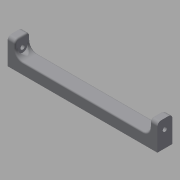
# Autodesk Inventor part: SwarmieLidSupport
Saved by Autodesk Inventor 2014 (Build 180170000, 170)
## iProperties
Created: 2015-05-25
Part Number: SwarmieLidSupport
Material: Generic
Document SubType Name: Modeling
Designer: Karl
Density: 1 g/cm^3
Appearance: Default
Author: Karl
Autodesk Inventor part; units mm, degrees
ref_plane "YZ Plane" through (0, 0, 0) normal (1, 0, 0) x (0, 1, 0)
ref_plane "XZ Plane" through (0, 0, 0) normal (0, 1, 0) x (-1, 0, 0)
ref_plane "XY Plane" through (0, 0, 0) normal (0, 0, 1) x (1, 0, 0)
sketch "Sketch1" plane through (0, 0, 0) normal (0, 1, 0) x (-1, 0, 0)
  line L0 (63.5, -6.35) -> (-63.5, -6.35)
  line L1 (-63.5, -6.35) -> (-63.5, 6.35)
  line L2 (-63.5, 6.35) -> (63.5, 6.35)
  line L3 (63.5, 6.35) -> (63.5, -6.35)
  line L4 (63.5, -6.35) -> (-63.5, 6.35) construction
  line L5 (-63.5, -6.35) -> (63.5, 6.35) construction
  point P0 (0, 0)
  dimension "d0" = 12.7
  dimension "d1" = 127
  constraints: 12 end point, 2 midpoint, 2 parallel, 1 horizontal, 1 perpendicular
  measures "d0" distance of L0.end L1.end
  measures "d1" distance of L1.end L2.end
extrude "Extrusion1" add sketch "Sketch1" along normal blind 22.225
sketch "Sketch2" plane through (-63.5, 0, 6.35) normal (0, 0, 1) x (1, 0, 0)
  line L0 (127, 0) -> (0, 0) projected
  line L1 (127, 0) -> (127, 22.225) projected
  line L2 (0, 22.225) -> (127, 22.225) projected
  line L3 (0, 0) -> (0, 22.225) projected
  line L4 (6.35, 22.225) -> (120.65, 22.225)
  line L5 (120.65, 22.225) -> (120.65, 9.525)
  line L6 (120.65, 9.525) -> (6.35, 9.525)
  line L7 (6.35, 9.525) -> (6.35, 22.225)
  point P0 (63.5, 0)
  dimension "d4" = 6.35
  dimension "d5" = 6.35
  dimension "d6" = 9.525
  constraints: 8 end point, 2 parallel, 1 horizontal, 1 perpendicular, 1 point on line
  measures "d4" distance between parallel lines of L3 L7
  measures "d5" distance between parallel lines of L1 L5
  measures "d6" distance between parallel lines of L0 L6
extrude "Extrusion2" cut sketch "Sketch2" against normal blind 22.225 contours L5 L6 L7 L2
fillet "Fillet1" radius 6.35 2 edges at (57.15, 9.525, 0) (-57.15, 9.525, 0)
sketch "Sketch3" plane through (-57.15, 22.225, 6.35) normal (1, 0, 0) x (0, 0, -1)
  line L0 (0, 0) -> (12.7, 0) projected
  point P0 (6.35, -22.225)
  point P1 (6.35, -8.255)
  dimension "d10" = 8.255
  constraints: 1 vertical alignment
  measures "d10" distance from line of point (6.35, -8.255) L0
hole "Hole1" at (-57.15, 13.97, 0) direction (-1, 0, 0) diameter 3.683 end through all
sketch "Sketch4" plane through (-63.5, 0, -6.35) normal (-1, 0, 0) x (0, 0, 1)
  circle A0 centre (6.35, 13.97) radius 1.8415 projected
  point P0 (6.35, 0)
  constraints: 1 coincident
hole "Hole2" at (-63.5, 13.97, 0) direction (1, 0, 0) diameter 3.683 end through all
sketch "Sketch5" plane through (57.15, 22.225, -6.35) normal (-1, 0, 0) x (0, 0, 1)
  circle A0 centre (6.35, -8.255) radius 1.8415 projected
  circle A1 centre (6.35, -8.255) radius 4.064
  point P0 (6.35, -22.225)
  dimension "d25" = 8.128
  constraints: 1 centre point, 1 coincident
  measures "d25" diameter of A1
extrude "Extrusion3" cut sketch "Sketch5" along normal blind 22.225
fillet "Fillet2" radius 3.175 4 edges at (60.325, 22.225, 6.35) (60.325, 22.225, -6.35) (-60.325, 22.225, 6.35) (-60.325, 22.225, -6.35)
sketch "Sketch6" plane through (-57.15, 15.875, 6.35) normal (1, 0, 0) x (0, 0, -1)
  circle A0 centre (6.35, -1.905) radius 1.8415 projected
  circle A1 centre (6.35, -1.905) radius 4.064
  point P0 (6.35, -15.875)
  dimension "d29" = 8.128
  constraints: 1 centre point, 1 coincident
  measures "d29" diameter of A1
extrude "Extrusion4" cut sketch "Sketch6" along normal blind 22.225
fillet "Fillet3" radius 1.27 16 edges at (-55.2901, 11.3849, 6.35) (-57.15, 17.4625, 6.35) (-57.15, 21.2951, 5.4201) (-57.15, 22.225, 0) (-57.15, 21.2951, -5.4201) (-57.15, 17.4625, -6.35) (-55.2901, 11.3849, -6.35) (0, 9.525, -6.35) (55.2901, 11.3849, -6.35) (57.15, 17.4625, -6.35) (57.15, 21.2951, -5.4201) (57.15, 22.225, 0) (57.15, 21.2951, 5.4201) (57.15, 17.4625, 6.35) (55.2901, 11.3849, 6.35) (0, 9.525, 6.35)
body "Solid1"
